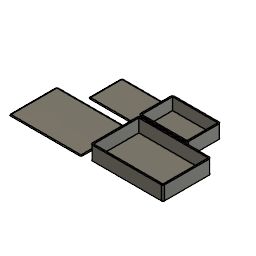
haptic_2BOX (Autodesk Fusion 360 design; units mm, degrees)
part number: 2026-03-26-10-40-11-151
Autodesk Fusion 360 part; units mm, degrees
sketch "스케치1" plane through (0, 0, 0) normal (0, 1, 0) x (1, 0, 0)
  line L0 (0, 0) -> (100, 0)
  line L1 (100, 0) -> (100, -70)
  line L2 (100, -70) -> (0, -70)
  line L3 (0, -70) -> (0, 0)
  dimension "d1" = 100
  dimension "d2" = 70
  constraint horizontal L0
  constraint vertical L1
  constraint horizontal L2
  constraint vertical L3
  constraint coincident L0.start L3.end
  measures "d1" distance of L0.start L0.end
  measures "d2" distance of L0.start L2.end
extrude "돌출1" add sketch "스케치1" along normal blind 28 makes body 1
shell "쉘1" thickness 3 removed faces 1 at (33.3333, 28, 23.3333) on bodies 1
sketch "스케치2" plane through (0, 3, 0) normal (0, 1, 0) x (-1, 0, 0)
  line L0 (-3, 67) -> (-97, 67)
  line L1 (-97, 67) -> (-97, 3)
  line L2 (-97, 3) -> (-3, 3)
  line L3 (-3, 3) -> (-3, 67)
  line L4 (5, 70) -> (105, 70)
  line L5 (105, 70) -> (105, 0)
  line L6 (105, 0) -> (5, 0)
  line L7 (5, 0) -> (5, 70)
  dimension "d8" = 100
  constraint horizontal L4
  constraint vertical L5
  constraint horizontal L6
  constraint vertical L7
  measures "d8" distance of L4.start L4.end
extrude "돌출2" add sketch "스케치2" along normal blind 1 separate body contours L4 L5 L6 L7 makes body 2
sketch "스케치4" plane through (0, 3, 0) normal (0, 1, 0) x (-1, 0, 0)
  line L0 (-3, 67) -> (-97, 67)
  line L1 (-97, 67) -> (-97, 3)
  line L2 (-97, 3) -> (-3, 3)
  line L3 (-3, 3) -> (-3, 67)
  line L4 (-225, 275) -> (-75, 275)
  line L5 (-75, 275) -> (-75, 175)
  line L6 (-75, 175) -> (-225, 175)
  line L7 (-225, 175) -> (-225, 275)
  dimension "d13" = 150
  dimension "d14" = 100
  constraint horizontal L4
  constraint vertical L5
  constraint horizontal L6
  constraint vertical L7
  measures "d13" distance of L4.start L4.end
  measures "d14" distance of L4.start L6.end
sketch "스케치5" plane through (0, 0, 0) normal (0, 1, 0) x (1, 0, 0)
  line L0 (50, -275) -> (-100, -275)
  line L1 (-100, -275) -> (-100, -375)
  line L2 (-100, -375) -> (50, -375)
  line L3 (50, -375) -> (50, -275)
  dimension "d15" = 150
  dimension "d16" = 100
  constraint horizontal L0
  constraint vertical L1
  constraint horizontal L2
  constraint vertical L3
  measures "d15" distance of L0.start L0.end
  measures "d16" distance of L0.start L2.end
extrude "돌출3" add sketch "스케치4" along normal blind 30 separate body contours L4 L5 L6 L7 makes body 3
shell "쉘2" thickness 3 removed faces 1 at (175, 33, 241.6667) on bodies 3
extrude "돌출4" add sketch "스케치5" along normal blind 1 separate body makes body 4
fillet "필렛5" radius 3 4 edges at (0, 14, 0) (100, 14, 0) (0, 14, 70) (100, 14, 70) on bodies 1
fillet "필렛7" radius 3 4 edges at (225, 18, 175) (225, 18, 275) (75, 18, 275) (75, 18, 175) on bodies 3
fillet "필렛8" radius 3 1 edges at (-100, 0.5, 275) on bodies 4
fillet "필렛9" radius 3 1 edges at (50, 0.5, 275) on bodies 4
fillet "필렛10" radius 3 1 edges at (50, 0.5, 375) on bodies 4
fillet "필렛11" radius 3 1 edges at (-100, 0.5, 375) on bodies 4
fillet "필렛12" radius 3 8 edges at (-99.1213, 1, 374.1213) (-25, 1, 375) (49.1213, 1, 374.1213) (50, 1, 325) (49.1213, 1, 275.8787) (-25, 1, 275) (-99.1213, 1, 275.8787) (-100, 1, 325) on bodies 4
fillet "필렛13" radius 3 3 edges at (-5, 3.5, 0) (-105, 3.5, 0) (-105, 3.5, 70) on bodies 2
fillet "필렛14" radius 3 1 faces at (-38.3333, 4, 46.6667) on bodies 2
fillet "필렛15" radius 1 1 faces at (126, 3, 208.3333) on bodies 3
move_body "이동1" bodies 4 to x (1, 0, 0) y (0, 1, 0) z (0, 0, 1) at (-55, 5, -190)
move_body "이동2" bodies 1 to x (1, 0, 0) y (0, 1, 0) z (0, 0, 1) at (0, 1, 0)
move_body "이동3" bodies 1 to x (1, 0, 0) y (0, 1, 0) z (0, 0, 1) at (0, 2, 0)
move_body "이동4" bodies 3 to x (1, 0, 0) y (0, 1, 0) z (0, 0, 1) at (-70, 0, -100)
move_body "이동5" bodies 3 1 to x (1, 0, 0) y (0, 1, 0) z (0, 0, 1) at (0, 5, 0)
move_body "이동6" bodies 4 2 to x (1, 0, 0) y (0, 1, 0) z (0, 0, 1) at (0, 10, 0)
